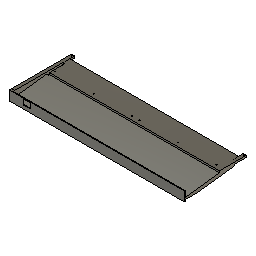
case-middle (Autodesk Fusion 360 design; units mm, degrees)
part number: 2025-12-05-02-40-18-396
Autodesk Fusion 360 part; units mm, degrees
note: some values were not read from the file. Set by a fixed rule: which sketch regions a step uses; the direction of a hole.
sketch "sketch-thing" plane through (0, 0, 0) normal (1, 0, 0) x (0, 1, 0)
  line L0 (0, 0) -> (-127.2538, 0)
  line L1 (-127.2538, -15.6248) -> (-127.2538, 6.9478)
  line L2 (-0.8531, 6.9478) -> (0, 6.9478)
  line L3 (0, 6.9478) -> (1.6, 6.9478)
  line L4 (-127.2538, 0) -> (-127.2538, -15.6248)
  line L5 (-0.0202, 0) -> (-127.2538, 0)
  line L6 (-127.2538, 6.9478) -> (-0.8531, 6.9478)
  line L7 (1.6, 0.1989) -> (-0.0202, 0)
  line L8 (1.6, 6.9478) -> (1.6, 0.1989)
  line L9 (-127.2538, -15.6248) -> (0, 0)
  line L10 (0, 0) -> (-0.8531, 6.9478)
  line L11 (-0.8531, 6.9478) -> (-127.2538, -8.5722)
  line L12 (0, 6.9478) -> (0, 0)
  line L13 (-127.1077, 3.7478) -> (0, 3.7478)
  line L14 (-127.2538, 0.7478) -> (-56.2538, 0.7478)
  line L15 (-127.2538, 6.9478) -> (-128.8538, 6.9478)
  line L16 (-128.8538, 6.9478) -> (-128.8538, -15.8213)
  line L17 (-127.2538, -15.6248) -> (-128.8538, -15.8213)
  line L18 (-0.6093, 4.9627) -> (-127.0101, -10.5573)
  line L19 (-87.2538, -3.6609) -> (-87.2538, 3.7478)
  line L20 (-56.2538, 3.7478) -> (-56.2538, 0.1455)
  line L21 (-127.1077, 3.7478) -> (-128.8538, 3.7478)
  line L22 (-24.433, -3) -> (-24.433, 0)
  line L23 (-127.2538, -8.5722) -> (-126.4008, -15.5201)
  line L24 (-127.2538, -8.5722) -> (-120.2538, -8.5722) construction
  line L25 (-126.7691, -12.5201) -> (-101.9677, -12.5201)
  dimension "d3" = 3.2
  dimension "d5" = 3
  dimension "d6" = 71
  dimension "d93" = 83
  dimension "d94" = 97
  dimension "d95" = 3
  constraint coincident L13 L20.start
  constraint coincident L11 L20.end
  constraint perpendicular L14 L20
  constraint coincident L16 L21.end
  constraint perpendicular L16 L21
  constraint vertical L22
  constraint coincident L0 L22.end
  constraint horizontal L24
  constraint coincident L9 L23.end
  constraint perpendicular L9 L23
  constraint coincident L23 L25.start
  constraint coincident L9 L25.end
  measures "d3" distance of L6 L13
  measures "d5" distance of L13 L14
  measures "d6" distance of L1 L20
  measures "d93" angle of L23 L24
  measures "d94" angle of L23 L25
  measures "d95" distance of L23.end L25
extrude "Extrude1" add sketch "sketch-thing" along normal blind 349.4 contours L0 L5 L11 L13 L18 | L0 L5 L11 L18 L23 | L11 L13 L20 | L1 L4 L9 L23 | L1 L4 L16 L17 L21
extrude "Extrude2" add sketch "sketch-thing" against normal blind 6.4 contours L0 L5 L7 L9 L10 L13 L18 | L0 L5 L9 L18 L22 L23 L25 | L0 L5 L11 L13 L18 | L0 L5 L11 L18 L23 | L11 L13 L20 | L0 L5 L11 L19 | L0 L5 L11 L14 L19 L20 | L1 L4 L9 L23 | L13 L14 L19 L20 | L0 L1 L4 L5 L11 L19 | L0 L1 L5 L14 L19 | L1 L4 L16 L17 L21 | L1 L13 L14 L19 L21
sketch "Sketch2" plane through (349.4, 0, 0) normal (1, 0, 0) x (0, 1, 0)
  line L0 (-56.2538, 3.7478) -> (-56.2538, 0.1455)
  line L1 (-56.2538, 0.1455) -> (-127.2538, -8.5722)
  line L2 (-127.2538, -8.5722) -> (-127.2538, 3.7478)
  line L3 (-10.504, 3.7478) -> (-56.2538, 3.7478)
  line L4 (-128.8538, 3.7478) -> (-128.8538, -15.8213)
  line L5 (-128.8538, -15.8213) -> (-126.4008, -15.5201)
  line L6 (-127.0101, -10.5573) -> (-10.504, 3.7478)
  line L7 (0, 0) -> (-128.8538, -15.8213)
  line L8 (-56.2538, 3.7478) -> (0, 3.7478)
  line L9 (0, 3.7478) -> (0, 0)
  line L10 (0, 0) -> (-0.4602, 3.7478)
  line L11 (-24.433, 3.7478) -> (-24.433, -3)
  line L12 (0, 0) -> (-24.433, 0)
  line L13 (-126.3318, -16.082) -> (-126.9165, -11.3197)
  line L14 (-126.7691, -12.5201) -> (-101.9677, -12.5201)
  line L15 (-126.4008, -15.5201) -> (-127.0101, -10.5573)
  line L16 (-127.2538, 3.7478) -> (-128.8538, 3.7478)
  dimension "d11" = 7
  dimension "d88" = 24.433
  dimension "d89" = 3
  constraint coincident L7.start L9.end
  constraint coincident L4.end L5.start
  constraint coincident L0.start L3.end
  constraint perpendicular L4 L8
  constraint perpendicular L8 L9
  constraint coincident L8 L10.end
  constraint coincident L8 L11.start
  constraint coincident L7 L11.end
  constraint perpendicular L8 L11
  constraint coincident L11 L12.end
  constraint perpendicular L11 L12
  constraint perpendicular L7 L13
  constraint horizontal L14
  constraint coincident L13 L14.start
  constraint coincident L7 L14.end
  measures "d11" angle of L9 L10
  measures "d88" distance of L9 L11
  measures "d89" distance of L5.end L14
extrude "Extrude3" add sketch "Sketch2" along normal blind 6.4 contours L0 L1 L2 L3 L4 L5 L6 L7 L8 L11 L13 L15 L16 | L3 L6 L8 L11 | L6 L8 L10 L11 L12 | L6 L7 L11 L13 L14 L15
sketch "Sketch3" plane through (0, 0, 0) normal (0, 0, 1) x (1, 0, 0)
  line L0 (0, 0) -> (355.8, 0)
  line L1 (355.8, 0) -> (355.8, -128.854)
  line L2 (355.8, -128.854) -> (0, -128.854)
  line L3 (0, -128.854) -> (0, 0)
  line L4 (0, 0) -> (-6.4, 0)
  line L5 (-6.4, 0) -> (-6.4, -128.854)
  line L6 (-6.4, -128.854) -> (0, -128.854)
  line L7 (0, -128.854) -> (0, 0)
  line L8 (0, -127.2538) -> (0, -0.8531)
  circle A0 centre (-3.2, -3.2) radius 1.1
  line L9 (349.4, -128.854) -> (349.4, 0)
  line L10 (0, -56.254) -> (349.4, -56.254)
  circle A1 centre (341.787, -48.641) radius 1.1
  line L11 (0, -41.028) -> (349.4, -41.028)
  line L12 (175, 0) -> (175, -128.854)
  line L13 (262.05, 0) -> (262.05, -128.854)
  circle A2 centre (262.05, -48.641) radius 1.1
  circle A3 centre (182.613, -48.641) radius 1.1
  circle A4 centre (167.387, -48.641) radius 1.1
  circle A5 centre (7.613, -48.641) radius 1.1
  circle A6 centre (87.65, -48.641) radius 1.1
  circle A7 centre (352.6, -3.2) radius 1.1
  circle A8 centre (352.6, -124.054) radius 1.1
  circle A9 centre (-3.2, -124.054) radius 1.1
  dimension "d14" = 355.8
  dimension "d15" = 128.854
  dimension "d16" = 6.4
  dimension "d17" = 2.2
  dimension "d18" = 3.2
  dimension "d19" = 3.2
  dimension "d20" = 6.4
  dimension "d21" = 72.6
  dimension "d22" = 2.2
  dimension "d23" = 7.613
  dimension "d24" = 41.028
  dimension "d25" = 7.613
  dimension "d26" = 174.4
  dimension "d27" = 87.35
  dimension "d28" = 2.2
  dimension "d29" = 7.613
  dimension "d30" = 2.2
  dimension "d31" = 7.613
  dimension "d32" = 7.613
  dimension "d33" = 2.2
  dimension "d34" = 7.613
  dimension "d35" = 7.613
  dimension "d36" = 2.2
  dimension "d37" = 7.613
  dimension "d38" = 7.613
  dimension "d39" = 2.2
  dimension "d40" = 87.35
  dimension "d71" = 7.613
  dimension "d77" = 2.2
  dimension "d78" = 3.2
  dimension "d79" = 3.2
  dimension "d80" = 2.2
  dimension "d81" = 3.2
  dimension "d82" = 4.8
  dimension "d83" = 2.2
  dimension "d84" = 3.2
  dimension "d85" = 4.8
  constraint horizontal L0
  constraint vertical L1
  constraint horizontal L2
  constraint vertical L3
  constraint coincident L0.start L3.end
  constraint horizontal L4
  constraint vertical L5
  constraint horizontal L6
  constraint vertical L7
  constraint coincident L2 L9.start
  constraint coincident L0 L9.end
  constraint perpendicular L0 L9
  constraint coincident L3 L10.start
  constraint coincident L9 L10.end
  constraint perpendicular L9 L10
  constraint coincident L7 L11.start
  constraint coincident L9 L11.end
  constraint perpendicular L9 L11
  constraint coincident L0 L12.start
  constraint coincident L2 L12.end
  constraint perpendicular L2 L12
  constraint coincident L0 L13.start
  constraint coincident L2 L13.end
  constraint perpendicular L2 L13
  constraint coincident L13 A2.centre
  measures "d14" distance of L0.start L0.end
  measures "d15" distance of L0.start L2.end
  measures "d16" distance of L5 L8
  measures "d17" diameter of A0
  measures "d18" distance of L5 A0.centre
  measures "d19" distance of L4 A0.centre
  measures "d20" distance of L1 L9
  measures "d21" distance of L2 L10
  measures "d22" diameter of A1
  measures "d23" distance of L10 A1.centre
  measures "d24" distance of L0 L11
  measures "d25" distance of L9 A1.centre
  measures "d26" distance of L9 L12
  measures "d27" distance of L9 L13
  measures "d28" diameter of A2
  measures "d29" distance of L11 A2.centre
  measures "d30" diameter of A3
  measures "d31" distance of L12 A3.centre
  measures "d32" distance of L11 A3.centre
  measures "d33" diameter of A4
  measures "d34" distance of L12 A4.centre
  measures "d35" distance of L11 A4.centre
  measures "d36" diameter of A5
  measures "d37" distance of L11 A5.centre
  measures "d38" distance of L8 A5.centre
  measures "d39" diameter of A6
  measures "d40" distance of L12 A6.centre
  measures "d71" distance of L11 A6.centre
  measures "d77" diameter of A7
  measures "d78" distance of L0 A7.centre
  measures "d79" distance of L1 A7.centre
  measures "d80" diameter of A8
  measures "d81" distance of L1 A8.centre
  measures "d82" distance of L2 A8.centre
  measures "d83" diameter of A9
  measures "d84" distance of L5 A9.centre
  measures "d85" distance of L6 A9.centre
hole "Hole1" at (7.613, -48.641, 0) direction (0, 0, -1) diameter 5 end through all
hole "Hole2" at (7.613, -48.641, 0) direction (0, 0, 1) diameter 2.2 end through all
hole "Hole5" at (167.387, -48.641, 0) direction (0, 0, -1) diameter 5 end through all
hole "Hole6" at (167.387, -48.641, 0) direction (0, 0, 1) diameter 2.2 end through all
hole "Hole7" at (182.613, -48.641, 0) direction (0, 0, -1) diameter 5 end through all
hole "Hole8" at (182.613, -48.641, 0) direction (0, 0, 1) diameter 2.2 end through all
hole "Hole9" at (262.05, -48.641, 0) direction (0, 0, -1) diameter 5 end through all
hole "Hole10" at (262.05, -48.641, 0) direction (0, 0, 1) diameter 2.2 end through all
hole "Hole11" at (341.787, -48.641, 0) direction (0, 0, -1) diameter 5 end through all
hole "Hole12" at (341.787, -48.641, 0) direction (0, 0, 1) diameter 2.2 end through all
hole "Hole13" at (87.65, -48.641, 0) direction (0, 0, -1) diameter 5 end through all
hole "Hole14" at (87.65, -48.641, 0) direction (0, 0, 1) diameter 2.2 end through all
hole "Hole15" at (352.6, -3.2, 0) direction (0, 0, 1) diameter 2.2 end through all
hole "Hole16" at (352.6, -124.054, 0) direction (0, 0, -1) diameter 2.2 end through all
hole "Hole17" at (352.6, -124.054, 0) direction (0, 0, 1) diameter 2.2 end through all
hole "Hole18" at (-3.2, -124.054, 0) direction (0, 0, -1) diameter 2.2 end through all
hole "Hole19" at (-3.2, -124.054, 0) direction (0, 0, 1) diameter 2.2 end through all
hole "Hole20" at (-3.2, -3.2, 0) direction (0, 0, 1) diameter 2.2 end through all
sketch "Sketch7" plane through (0, -0.6093, 4.9627) normal (0, 0.121869, -0.992546) x (-1, 0, 0)
  ellipse E0 centre (-87.65, -48.3924) end of major axis (-87.65, -50.9111) minor radius 2.5
  ellipse E1 centre (-341.787, -48.3924) end of major axis (-341.787, -50.9111) minor radius 2.5
  ellipse E2 centre (-262.05, -48.3924) end of major axis (-262.05, -50.9111) minor radius 2.5
  ellipse E3 centre (-182.613, -48.3924) end of major axis (-182.613, -50.9111) minor radius 2.5
  ellipse E4 centre (-167.387, -48.3924) end of major axis (-167.387, -50.9111) minor radius 2.5
  ellipse E5 centre (-7.613, -48.3924) end of major axis (-7.613, -50.9111) minor radius 2.5
  line L0 (0, -9.9689) -> (-349.4, -9.9689)
  line L1 (-349.4, -9.9689) -> (-349.4, -127.35)
  line L2 (-349.4, -127.35) -> (0, -127.35)
  line L3 (0, -127.35) -> (-349.4, -127.35)
  line L4 (-349.4, -127.35) -> (-349.4, -9.9689)
  line L5 (-349.4, -9.9689) -> (0, -9.9689)
  line L6 (0, -9.9689) -> (0, -127.35)
  line L7 (-4, -9.9689) -> (-4, -127.35)
  line L8 (0, -34.55) -> (-4, -34.55)
  line L9 (0, -23.55) -> (-4, -23.55)
  line L10 (0, -57) -> (-4, -57)
  line L11 (0, -127.35) -> (0, -9.9689)
  dimension "d109" = 4
  dimension "d110" = 92.8
  dimension "d111" = 11
  constraint horizontal L3
  constraint vertical L4
  constraint horizontal L5
  constraint vertical L6
  constraint coincident L0.end L1.start
  constraint coincident L2.end L3.start
  constraint coincident L5 L7.start
  constraint coincident L3 L7.end
  constraint perpendicular L3 L7
  constraint coincident L6 L8.start
  constraint coincident L7 L8.end
  constraint perpendicular L7 L8
  constraint coincident L6 L9.start
  constraint coincident L7 L9.end
  constraint perpendicular L7 L9
  constraint coincident L6 L10.start
  constraint coincident L7 L10.end
  constraint perpendicular L7 L10
  measures "d109" distance of L6 L7
  measures "d110" distance of L3 L8
  measures "d111" distance of L8 L9
extrude "Extrude4" cut sketch "Sketch7" against normal blind 10 contours L6 L7 L8 L9 L11 | L6 L7 L8 L10 L11
sketch "Sketch8" plane through (0, -127.2538, 0) normal (0, 1, 0) x (-1, 0, 0)
  line L0 (0, 3.7478) -> (-355.8, 3.7478)
  line L1 (-355.8, -8.5722) -> (0, -8.5722)
  line L2 (0, -8.5722) -> (-355.8, -8.5722)
  line L3 (-22.005, -8.5722) -> (-22.005, 2.4278)
  line L4 (-37.005, -8.5722) -> (-37.005, 2.4278)
  line L5 (-37.005, 2.4278) -> (-22.005, 2.4278)
  line L6 (0, -8.5722) -> (0, 3.7478)
  line L7 (-355.8, 3.7478) -> (-355.8, -8.5722)
  dimension "d114" = 22.005
  dimension "d115" = 15
  dimension "d116" = 11
  constraint coincident L1.end L2.start
  constraint coincident L1.start L2.end
  constraint coincident L2 L3.start
  constraint perpendicular L0 L3
  constraint coincident L2 L4.start
  constraint perpendicular L2 L4
  constraint coincident L4 L5.start
  constraint coincident L3 L5.end
  constraint perpendicular L3 L5
  measures "d114" distance of L1.end L3
  measures "d115" distance of L3 L4
  measures "d116" distance of L2 L5
extrude "Extrude5" cut sketch "Sketch8" against normal blind 5 contours L1 L2 L3 L4 L5
